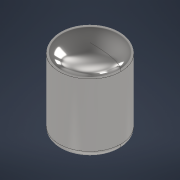
# Autodesk Inventor part: fuel tank
Saved by Autodesk Inventor 2021 (Build 250183000, 183)
## iProperties
Created: 2020-12-01
Part Number: fuel tank
Material: Stainless Steel
Document SubType Name: Modeling
Designer: henry
Density: 8 g/cm^3
Appearance: Semi-Polished
Author: henry
Autodesk Inventor part; units mm, degrees
ref_plane "YZ Plane" through (0, 0, 0) normal (1, 0, 0) x (0, 1, 0)
ref_plane "XZ Plane" through (0, 0, 0) normal (0, 1, 0) x (-1, 0, 0)
ref_plane "XY Plane" through (0, 0, 0) normal (0, 0, 1) x (1, 0, 0)
sketch "wall sketch" plane through (0, 0, 0) normal (0, 1, 0) x (-1, 0, 0)
  circle A0 centre (0, 0) radius 32
  circle A1 centre (0, 0) radius 30
  dimension "d1" = 2
  dimension "d4" = 60
  constraints: 2 centre point, 2 coincident
  measures "d1" radial gap between concentric circles of A0 A1
  measures "d4" diameter of A1
extrude "wall extrude" add sketch "wall sketch" along normal blind 65
sketch "bottom cap sketch" plane through (0, 0, 0) normal (0, 0, 1) x (1, 0, 0)
  line L0 (32, 0) -> (32, 65) projected
  line L1 (0, -10) -> (0, -8)
  spline S0 degree 4 poles (32, 0) (32, -6.9332) (24.0966, -9.0238) (10.4609, -10) (0, -10) knots 0 0 0 0 0 1 1 1 1 1
  line L2 (30, 0) -> (32, 0)
  line L3 (0, -8) -> (0, 0) construction
  line L4 (0, -29.9402) -> (0, 80.8234) projected
  spline S1 degree 5 poles (30, 0) (29.9988, -0.5683) (29.9375, -1.1354) (29.7754, -1.6987) (29.1539, -2.8371) (28.1635, -3.6826) (27.5666, -4.0714) (26.0046, -4.9187) (24.3241, -5.5071) (23.3036, -5.8072) (20.9706, -6.3862) (18.6026, -6.797) (17.2773, -6.9901) (14.4825, -7.3362) (11.6765, -7.5776) (10.2029, -7.682) (7.2793, -7.8502) (4.3527, -7.949) (2.9019, -7.9822) (1.451, -8) (0, -8) knots 0 0 0 0 0 0 0.085992 0.085992 0.085992 0.193381 0.193381 0.193381 0.354299 0.354299 0.354299 0.556879 0.556879 0.556879 0.780422 0.780422 0.780422 1 1 1 1 1 1
  point P0 (26, -7)
  dimension "d12" = 2
  dimension "d5" = 10
  dimension "d9" = 26
  dimension "d10" = 3
  constraints: 6 end point, 4 vertical, 1 coincident, 1 horizontal, 6 other
  measures "d5" distance of L1.start L3.end
  measures "d9" horizontal distance of L1.start point (26, -7)
  measures "d10" vertical distance of L1.start point (26, -7)
revolve "bottom cap revolution" add sketch "bottom cap sketch" angle 360 about axis through (0, -10, 0) along (0, 1, 0) separate body
ref_plane "middle plane" through (0, 32.5, 0) normal (0, 1, 0) x (1, 0, 0)
mirror "copy the cap up top" about plane through (0, 32.5, 0) normal (0, 1, 0) bodies 2 separate body
